Autodesk Inventor part; units mm, degrees
(part 2 of 2)
sketch "Sketch3" plane through (0, 0, 5.08) normal (0, 0, 1) x (1, 0, 0)
  circle A0 centre (-28.882, 46.0869) radius 2.2578
  circle A1 centre (37.3983, -26.6388) radius 2.2578
  circle A2 centre (60.018, 46.0869) radius 2.2578
  circle A3 centre (-67.2215, -66.8519) radius 2.2578
  circle A4 centre (60.018, 46.0869) radius 2.2578
  circle A5 centre (-28.882, 46.0869) radius 2.2578
  circle A6 centre (37.3983, -26.6388) radius 2.2578
  line L0 (-31.282, 2.4932) -> (-31.282, -13.5068) projected
  line L1 (-31.282, -13.5068) -> (-13.782, -13.5068) projected
  line L2 (-13.782, -13.5068) -> (-13.782, 2.4932) projected
  line L3 (-13.782, 2.4932) -> (-31.282, 2.4932) projected
  line L4 (24.318, -6.3631) -> (24.318, 9.6369) projected
  line L5 (24.318, 9.6369) -> (6.818, 9.6369) projected
  line L6 (6.818, 9.6369) -> (6.818, -6.3631) projected
  line L7 (6.818, -6.3631) -> (24.318, -6.3631) projected
  line L8 (44.918, -4.6506) -> (44.918, -20.6506) projected
  line L9 (44.918, -20.6506) -> (62.418, -20.6506) projected
  line L10 (62.418, -20.6506) -> (62.418, -4.6506) projected
  line L11 (62.418, -4.6506) -> (44.918, -4.6506) projected
  line L12 (43.368, -11.1256) -> (43.368, 4.8744) projected
  line L13 (43.368, 4.8744) -> (25.868, 4.8744) projected
  line L14 (25.868, 4.8744) -> (25.868, -11.1256) projected
  line L15 (25.868, -11.1256) -> (43.368, -11.1256) projected
  line L16 (5.268, -11.1256) -> (5.268, 4.8744) projected
  line L17 (5.268, 4.8744) -> (-12.232, 4.8744) projected
  line L18 (-12.232, 4.8744) -> (-12.232, -11.1256) projected
  line L19 (-12.232, -11.1256) -> (5.268, -11.1256) projected
  line L20 (43.368, 7.9244) -> (43.368, 23.9244) projected
  line L21 (43.368, 23.9244) -> (25.868, 23.9244) projected
  line L22 (25.868, 23.9244) -> (25.868, 7.9244) projected
  line L23 (25.868, 7.9244) -> (43.368, 7.9244) projected
  line L24 (24.318, 12.6869) -> (24.318, 28.6869) projected
  line L25 (24.318, 28.6869) -> (6.818, 28.6869) projected
  line L26 (6.818, 28.6869) -> (6.818, 12.6869) projected
  line L27 (6.818, 12.6869) -> (24.318, 12.6869) projected
  line L28 (44.918, 14.3994) -> (44.918, -1.6006) projected
  line L29 (44.918, -1.6006) -> (62.418, -1.6006) projected
  line L30 (62.418, -1.6006) -> (62.418, 14.3994) projected
  line L31 (62.418, 14.3994) -> (44.918, 14.3994) projected
  line L32 (5.268, 7.9244) -> (5.268, 23.9244) projected
  line L33 (5.268, 23.9244) -> (-12.232, 23.9244) projected
  line L34 (-12.232, 23.9244) -> (-12.232, 7.9244) projected
  line L35 (-12.232, 7.9244) -> (5.268, 7.9244) projected
  line L36 (-31.282, 21.5432) -> (-31.282, 5.5432) projected
  line L37 (-31.282, 5.5432) -> (-13.782, 5.5432) projected
  line L38 (-13.782, 5.5432) -> (-13.782, 21.5432) projected
  line L39 (-13.782, 21.5432) -> (-31.282, 21.5432) projected
  line L40 (43.368, 26.9744) -> (43.368, 42.9744) projected
  line L41 (43.368, 42.9744) -> (25.868, 42.9744) projected
  line L42 (25.868, 42.9744) -> (25.868, 26.9744) projected
  line L43 (25.868, 26.9744) -> (43.368, 26.9744) projected
  line L44 (24.318, 31.7369) -> (24.318, 47.7369) projected
  line L45 (24.318, 47.7369) -> (6.818, 47.7369) projected
  line L46 (6.818, 47.7369) -> (6.818, 31.7369) projected
  line L47 (6.818, 31.7369) -> (24.318, 31.7369) projected
  line L48 (44.918, 33.4494) -> (44.918, 17.4494) projected
  line L49 (44.918, 17.4494) -> (62.418, 17.4494) projected
  line L50 (62.418, 17.4494) -> (62.418, 33.4494) projected
  line L51 (62.418, 33.4494) -> (44.918, 33.4494) projected
  line L52 (5.268, 26.9744) -> (5.268, 42.9744) projected
  line L53 (5.268, 42.9744) -> (-12.232, 42.9744) projected
  line L54 (-12.232, 42.9744) -> (-12.232, 26.9744) projected
  line L55 (-12.232, 26.9744) -> (5.268, 26.9744) projected
  line L56 (-31.282, 40.5932) -> (-31.282, 24.5932) projected
  line L57 (-31.282, 24.5932) -> (-13.782, 24.5932) projected
  line L58 (-13.782, 24.5932) -> (-13.782, 40.5932) projected
  line L59 (-13.782, 40.5932) -> (-31.282, 40.5932) projected
  line L60 (-36.0267, -22.4786) -> (-30.7679, -37.5897) projected
  line L61 (-30.7679, -37.5897) -> (-14.2402, -31.8379) projected
  line L62 (-14.2402, -31.8379) -> (-19.4989, -16.7268) projected
  line L63 (-19.4989, -16.7268) -> (-36.0267, -22.4786) projected
  line L64 (-70.5257, -57.1358) -> (-57.0218, -65.7174) projected
  line L65 (-57.0218, -65.7174) -> (-47.6357, -50.9475) projected
  line L66 (-47.6357, -50.9475) -> (-61.1396, -42.3659) projected
  line L67 (-61.1396, -42.3659) -> (-70.5257, -57.1358) projected
  line L68 (12.5349, -16.7268) -> (7.2762, -31.8379) projected
  line L69 (7.2762, -31.8379) -> (23.804, -37.5897) projected
  line L70 (23.804, -37.5897) -> (29.0627, -22.4786) projected
  line L71 (29.0627, -22.4786) -> (12.5349, -16.7268) projected
  line L72 (-12.232, -15.4985) -> (-12.232, -31.4985) projected
  line L73 (-12.232, -31.4985) -> (5.268, -31.4985) projected
  line L74 (5.268, -31.4985) -> (5.268, -15.4985) projected
  line L75 (5.268, -15.4985) -> (-12.232, -15.4985) projected
  line L76 (-56.2053, -36.8915) -> (-46.2721, -49.4347) projected
  line L77 (-46.2721, -49.4347) -> (-32.553, -38.5703) projected
  line L78 (-32.553, -38.5703) -> (-42.4861, -26.0271) projected
  line L79 (-42.4861, -26.0271) -> (-56.2053, -36.8915) projected
  arc A7 (66.368, 46.0869) -> (60.018, 52.4369) centre (60.018, 46.0869) ccw projected
  line L80 (66.368, 46.0869) -> (66.368, -19.3337) projected
  arc A8 (60.6824, -25.6489) -> (66.368, -19.3337) centre (60.018, -19.3337) ccw projected
  arc A9 (60.6824, -25.6489) -> (29.0899, -40.1547) centre (66.368, -79.6875) ccw projected
  arc A10 (22.0394, -41.2849) -> (29.0899, -40.1547) centre (24.7335, -35.5347) ccw projected
  arc A11 (22.0394, -41.2849) -> (-55.1736, -71.5721) centre (-2.2075, -93.0363) ccw projected
  arc A12 (-76.6111, -57.9488) -> (-55.1736, -71.5721) centre (-63.4241, -60.8763) ccw projected
  arc A13 (-39.5057, -16.3259) -> (-76.6111, -57.9488) centre (-20.8194, -70.3346) ccw projected
  arc A14 (-39.5057, -16.3259) -> (-35.232, -10.3249) centre (-41.582, -10.3249) ccw projected
  line L81 (-35.232, -10.3249) -> (-35.232, 46.0869) projected
  arc A15 (-28.882, 52.4369) -> (-35.232, 46.0869) centre (-28.882, 46.0869) ccw projected
  line L82 (-28.882, 52.4369) -> (60.018, 52.4369) projected
  circle A16 centre (-67.2215, -66.8519) radius 2.2578 projected
  circle A17 centre (37.3983, -26.6388) radius 2.2578 projected
  circle A18 centre (60.018, 46.0869) radius 2.2578 projected
  circle A19 centre (-28.882, 46.0869) radius 2.2578 projected
  point P0 (0, 0)
  constraints: 14 concentric, 7 centre point
extrude "Extrusion3" cut sketch "Sketch3" against normal blind 25.4 contours A0 | A1 | A2 | A3
sketch "Sketch4" plane through (0, 0, 5.08) normal (0, 0, 1) x (1, 0, 0)
  arc A0 (-41.582, 38.9432) -> (-41.582, 26.2432) centre (-41.582, 32.5932) ccw projected
  arc A1 (-35.232, 19.8932) -> (-41.582, 26.2432) centre (-41.582, 19.8932) ccw projected
  arc A2 (-41.582, 38.9432) -> (-35.232, 45.2932) centre (-41.582, 45.2932) ccw projected
  circle A3 centre (-41.582, 32.5932) radius 2.7027 projected
  arc A4 (-74.3688, -36.8027) -> (-79.9706, -48.1295) centre (-77.7389, -42.1846) ccw projected
  arc A5 (-74.3688, -36.8027) -> (-65.9808, -35.3121) centre (-70.9987, -31.4208) ccw projected
  circle A6 centre (-77.7389, -42.1846) radius 2.7027 projected
  arc A7 (-76.064, -55.7004) -> (-79.9706, -48.1295) centre (-82.2023, -54.0744) ccw projected
  arc A8 (72.718, 0.0494) -> (72.718, 12.7494) centre (72.718, 6.3994) ccw projected
  arc A9 (66.368, 19.0994) -> (72.718, 12.7494) centre (72.718, 19.0994) ccw projected
  circle A10 centre (72.718, 6.3994) radius 2.7027 projected
  arc A11 (72.718, 0.0494) -> (66.368, -6.3006) centre (72.718, -6.3006) ccw projected
  line L0 (66.368, 19.0994) -> (66.368, -6.3006)
  line L1 (66.368, 46.0869) -> (66.368, -19.3337) projected
  line L2 (-35.232, 45.2932) -> (-35.232, 19.8932)
  line L3 (-35.232, -10.3249) -> (-35.232, 46.0869) projected
  arc A12 (-65.9808, -35.3121) -> (-76.064, -55.7004) centre (-20.8194, -70.3346) ccw
  arc A13 (-39.5057, -16.3259) -> (-76.6111, -57.9488) centre (-20.8194, -70.3346) ccw projected
  point P0 (0, 0)
  constraints: 4 end point, 2 collinear, 2 point on circle, 2 tangent, 1 centre point, 1 concentric, 1 other
extrude "Extrusion4" add sketch "Sketch4" against normal blind 5.08
thread "Thread1" size "1/4-20 UNC" class "2B" standard "ANSI Unified Screw Threads" full length
thread "Thread2" size "1/4-20 UNC" class "2B" standard "ANSI Unified Screw Threads" full length
thread "Thread3" size "1/4-20 UNC" class "2B" standard "ANSI Unified Screw Threads" full length
body "Solid1"
